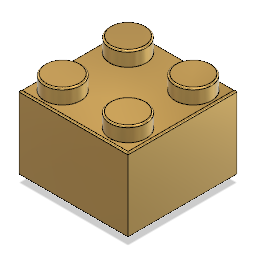
block v1 (Autodesk Fusion 360 design; units mm, degrees)
Autodesk Fusion 360 part; units mm, degrees
note: some values were not read from the file. Set by a fixed rule: which sketch regions a step uses.
sketch "Sketch1" plane through (0, 0, 0) normal (0, 1, 0) x (1, 0, 0) in component "block"
  line L0 (0, 0) -> (15, 0)
  line L1 (15, 0) -> (15, 15)
  line L2 (15, 15) -> (0, 15)
  line L3 (0, 15) -> (0, 0)
  dimension "d1" = 15
  dimension "d2" = 15
  constraint horizontal L0
  constraint vertical L1
  constraint horizontal L2
  constraint vertical L3
  constraint coincident L0.start L3.end
  measures "d1" distance of L0.start L0.end
  measures "d2" distance of L0.start L2.end
extrude "Extrude1" add sketch "Sketch1" along normal blind 10 in component "block"
sketch "Sketch2" plane through (0, 10, 0) normal (0, 1, 0) x (-1, 0, 0) in component "block"
  line L0 (0, -15) -> (0, 0)
  line L1 (0, 0) -> (-15, 0)
  line L2 (-15, 0) -> (-15, -15)
  line L3 (-15, -15) -> (0, -15)
  circle A0 centre (-3, -12) radius 2.5
  dimension "d5" = 5
  dimension "d6" = 3
  dimension "d7" = 3
  measures "d5" diameter of A0
  measures "d6" distance of L3 A0.centre
  measures "d7" distance of L0 A0.centre
extrude "Extrude2" add sketch "Sketch2" along normal blind 2 contours A0 in component "block"
pattern_linear "R-Pattern1" count 2 spacing 9 along (1, 0, 0) count 2 spacing 9 along (0, 0, 1) of "Extrude2" in component "block"
shell "Shell1" thickness 1 removed faces 1 at (5, 0, -10) in component "block"
sketch "Sketch3" plane through (0, 9, 0) normal (0, -1, 0) x (1, 0, 0) in component "block"
  circle A0 centre (12, -3) radius 1.5
  circle A1 centre (3, -3) radius 1.5
  circle A2 centre (12, -12) radius 1.5
  circle A3 centre (3, -12) radius 1.5
  line L0 (1, -1) -> (1, -14)
  line L1 (1, -14) -> (14, -14)
  line L2 (14, -14) -> (14, -1)
  line L3 (14, -1) -> (1, -1)
  line L4 (3, -3) -> (12, -12)
  circle A4 centre (7.5, -7.5) radius 3.5
  circle A5 centre (7.5, -7.5) radius 2.5
  dimension "d15" = 7
  dimension "d16" = -1
  constraint coincident A1.centre L4.start
  constraint coincident A2.centre L4.end
  constraint midpoint L4 A4.centre
  measures "d15" diameter of A4
extrude "Extrude3" add sketch "Sketch3" along normal blind 10 contours L4 A4 A5 | L4 A4 A5 in component "block"
fillet "Fillet1" radius 0.2 8 edges at (5.3308, 12, -3.904) (5.3308, 12, -12.904) (14.3308, 12, -12.904) (14.3308, 12, -3.904) (7.5, 10, 0) (15, 10, -7.5) (7.5, 10, -15) (0, 10, -7.5) in component "block"
component "block" placed x (1, 0, 0) y (0, 1, 0) z (0, 0, 1) at (0, 0, 0)
